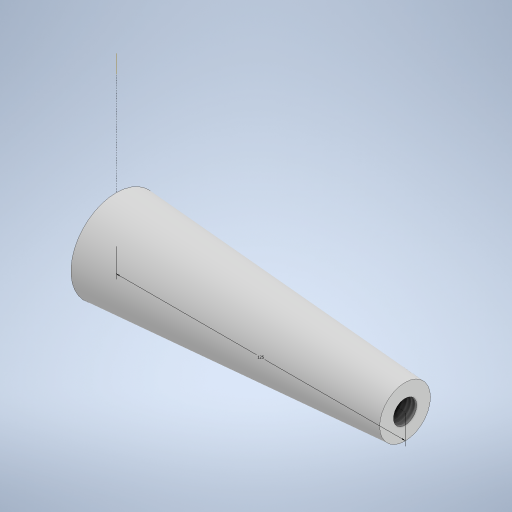
# Autodesk Inventor part: 10_Manija
Saved by Autodesk Inventor 2024.2 (Build 282272000, 272)
## iProperties
Created: 2024-04-26
Part Number: 10_Manija
Material: Genérico
Document SubType Name: Modeling
Designer: Cosmic Dinodog
Density: 1 g/cm^3
Appearance: Valor por defecto
Author: Cosmic Dinodog
Autodesk Inventor part; units mm, degrees
ref_plane "YZ Plane" through (0, 0, 0) normal (1, 0, 0) x (0, 1, 0)
ref_plane "XZ Plane" through (0, 0, 0) normal (0, 1, 0) x (-1, 0, 0)
ref_plane "XY Plane" through (0, 0, 0) normal (0, 0, 1) x (1, 0, 0)
sketch "Boceto1" plane through (0, 0, 0) normal (1, 0, 0) x (0, 1, 0)
  circle A0 centre (0, 0) radius 11
  dimension "d0" = 22
  constraints: 1 centre point, 1 coincident
  measures "d0" diameter of A0
sketch "Boceto2" plane through (0, 0, 0) normal (0, 0, 1) x (1, 0, 0)
  line L0 (0, 0) -> (-125, 0) construction
  line L1 (-125, 0) -> (-125, 64.0016) construction
  dimension "d1" = 125
  constraints: 4 end point, 1 horizontal, 1 vertical
  measures "d1" distance of L0.start L0.end
ref_plane "Plano de trabajo1" through (-125, 0, 0) normal (-1, 0, 0) x (0, -1, 0)
sketch "Boceto3" plane through (-125, 0, 0) normal (-1, 0, 0) x (0, -1, 0)
  circle A0 centre (0, 0) radius 19.614
  dimension "d2" = 39.228
  constraints: 1 centre point, 1 coincident
  measures "d2" diameter of A0
loft "Solevación1" add profiles "Boceto3", "Boceto1"
sketch "Boceto4" plane through (0, 0, 0) normal (0, 0, 1) x (1, 0, 0)
  line L0 (-125, -19.614) -> (-125, 19.614) projected
  arc A0 (-125, 19.614) -> (-129.0077, 0) centre (-79.0077, 0) ccw
  line L1 (-125, 19.614) -> (-125, 0)
  line L2 (-129.0077, 0) -> (-125, 0)
  line L3 (-125, 0) -> (-125, 19.614)
  point P0 (0, 0)
  dimension "d8" = 50
  constraints: 6 end point, 2 point on circle, 1 centre point, 1 collinear, 1 horizontal, 1 midpoint
  measures "d8" radius of A0
revolve "Revolución1" add sketch "Boceto4" angle 360 about axis through (-129.0077, 0, 0) along (1, 0, 0)
sketch "Boceto5" plane through (0, 0, 0) normal (1, 0, 0) x (0, 0, -1)
  point P0 (0, 0)
  point P1 (0, 0)
  constraints: 1 coincident
hole "Agujero1" at (0, 0, 0) direction (-1, 0, 0) diameter 10.106 depth 51 thread size "M12x1.75" class "6H" standard "ISO Metric profile"
